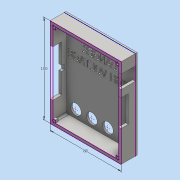
# Autodesk Inventor part: ATX Cover
Saved by Autodesk Inventor 2016 (Build 200138000, 138)
## iProperties
Created: 2016-08-04
Part Number: ATX Cover
Material: Generic
Document SubType Name: Modeling
Designer: Sam
Density: 1 g/cm^3
Appearance: Default
Author: Sam
Autodesk Inventor part; units mm, degrees
ref_plane "YZ Plane" through (0, 0, 0) normal (1, 0, 0) x (0, 1, 0)
ref_plane "XZ Plane" through (0, 0, 0) normal (0, 1, 0) x (-1, 0, 0)
ref_plane "XY Plane" through (0, 0, 0) normal (0, 0, 1) x (1, 0, 0)
sketch "Sketch1" plane through (0, 0, 0) normal (0, 1, 0) x (-1, 0, 0)
  line L0 (0, 0) -> (80, 0)
  line L1 (80, 0) -> (80, -100)
  line L2 (80, -100) -> (0, -100)
  line L3 (0, -100) -> (0, 0)
  line L4 (77, -97) -> (77, -3)
  line L5 (77, -3) -> (3, -3)
  line L6 (3, -3) -> (3, -97)
  line L7 (3, -97) -> (77, -97)
  line L8 (77, -3) -> (74, -3)
  line L9 (74, -3) -> (74, -6)
  line L10 (74, -6) -> (77, -6)
  line L11 (77, -6) -> (77, -3)
  line L12 (3, -3) -> (6, -3)
  line L13 (6, -3) -> (6, -6)
  line L14 (6, -6) -> (3, -6)
  line L15 (3, -6) -> (3, -3)
  line L16 (3, -97) -> (6, -97)
  line L17 (6, -97) -> (6, -94)
  line L18 (6, -94) -> (3, -94)
  line L19 (3, -94) -> (3, -97)
  line L20 (77, -97) -> (74, -97)
  line L21 (74, -97) -> (74, -94)
  line L22 (74, -94) -> (77, -94)
  line L23 (77, -94) -> (77, -97)
  point P0 (4, -4)
  point P1 (76, -4)
  point P2 (76, -96)
  point P3 (4, -96)
  dimension "d2" = 80
  dimension "d3" = 100
  constraints: 48 end point, 12 parallel, 6 perpendicular, 5 horizontal, 4 point on line, 3 other
  measures "d2" distance of L1.end L2.end
  measures "d3" distance of L0.end L1.end
extrude "Extrusion1" add sketch "Sketch1" along normal blind 16
extrude "Extrusion2" add sketch "Sketch1" along normal blind 3 contours L7 L21 L22 L4 | L10 L9 L5 L4 | L7 L6 L18 L17 | L13 L14 L6 L5
hole "Hole1" at (-4, 0, -4) at (-76, 0, -4) at (-76, 0, -96) at (-4, 0, -96) direction (0, 1, 0) diameter 3 end through all
sketch "Sketch2" plane through (0, 16, 0) normal (0, 1, 0) x (1, 0, 0)
  line L0 (-80, 0) -> (-80, 100) projected
  line L1 (-80, 0) -> (0, 0)
  line L2 (0, 0) -> (0, 100)
  line L3 (0, 100) -> (-80, 100)
  line L4 (-80, 100) -> (-80, 0)
  point P0 (-13, 89.5)
  point P1 (-31, 88)
  point P2 (-49, 88)
  point P3 (-67, 88)
  constraints: 8 end point, 2 parallel, 1 horizontal, 1 perpendicular
extrude "Extrusion3" add sketch "Sketch2" along normal blind 2
hole "Hole2" at (-67, 16, -88) at (-49, 16, -88) at (-31, 16, -88) at (-13, 16, -89.5) direction (0, 1, 0) diameter 12 end through all
sketch "Sketch3" plane through (0, 0, 0) normal (1, 0, 0) x (0, 0, -1)
  line L0 (94, 0) -> (6, 0) projected
  line L1 (5.118, 16) -> (94.882, 16) projected
  line L2 (12, 0) -> (27, 0)
  line L3 (27, 0) -> (27, 16)
  line L4 (27, 16) -> (12, 16)
  line L5 (12, 16) -> (12, 0)
  line L6 (35, 0) -> (65, 0)
  line L7 (65, 0) -> (65, 8)
  line L8 (65, 8) -> (35, 8)
  line L9 (35, 8) -> (35, 0)
  point P0 (0, 0)
  constraints: 16 end point, 4 parallel, 3 point on line, 2 horizontal, 2 perpendicular
extrude "Extrusion4" cut sketch "Sketch3" against normal blind 4
sketch "Sketch4" plane through (-80, 0, -100) normal (-1, 0, 0) x (0, 0, 1)
  line L0 (0, 0) -> (35, 0) projected
  line L1 (24, 0) -> (76, 0)
  line L2 (76, 0) -> (76, 10)
  line L3 (24, 10) -> (24, 0)
  line L4 (53, 10) -> (53, 13)
  line L5 (53, 13) -> (47, 13)
  line L6 (47, 13) -> (47, 10)
  line L7 (76, 10) -> (53, 10)
  line L8 (47, 10) -> (24, 10)
  point P0 (100, 0)
  constraints: 16 end point, 4 parallel, 1 horizontal, 1 perpendicular, 1 point on line
extrude "Extrusion5" cut sketch "Sketch4" against normal blind 4
sketch "Sketch5" plane through (0, 18, 0) normal (0, 1, 0) x (1, 0, 0)
  line L0 (0, 100) -> (-80, 100) projected
  line L1 (-80, 100) -> (-80, 0) projected
  line L2 (-80, 0) -> (0, 0) projected
  line L3 (0, 0) -> (0, 100) projected
  line L4 (-4, 20.3014) -> (-76, 20.3014) construction
  line L5 (-76, 20.3014) -> (-76, 40.6028) construction
  line L6 (-76, 40.6028) -> (-4, 40.6028) construction
  line L7 (-4, 40.6028) -> (-4, 20.3014) construction
  spline S0 degree 2 poles (-26.9997, 24.2223) (-26.9997, 25.2577) (-26.1604, 26.9241) (-25.4559, 27.3897) knots 0 0 0 1 2 2 2
  spline S1 degree 2 poles (-25.4559, 27.3897) (-24.88, 27.7511) (-23.6976, 27.9962) (-22.7786, 27.9962) knots 0 0 0 1 2 2 2
  line L8 (-22.7786, 27.9962) -> (-21.0387, 27.9962)
  line L9 (-21.0387, 27.9962) -> (-21.0387, 20.4362)
  line L10 (-21.0387, 20.4362) -> (-22.7603, 20.4362)
  spline S2 degree 2 poles (-22.7603, 20.4362) (-23.8263, 20.4362) (-25.0393, 20.7548) (-25.4681, 21.0366) knots 0 0 0 1 2 2 2
  spline S3 degree 2 poles (-25.4681, 21.0366) (-26.1972, 21.5206) (-26.9997, 23.1196) (-26.9997, 24.2223) knots 0 0 0 1 2 2 2
  spline S4 degree 2 poles (-25.9521, 24.2101) (-25.9521, 23.3401) (-25.3762, 22.1087) (-24.8065, 21.7595) knots 0 0 0 1 2 2 2
  spline S5 degree 2 poles (-24.8065, 21.7595) (-24.4021, 21.5206) (-23.4893, 21.3061) (-22.8093, 21.3061) knots 0 0 0 1 2 2 2
  line L11 (-22.8093, 21.3061) -> (-22.0435, 21.3061)
  line L12 (-22.0435, 21.3061) -> (-22.0435, 27.1262)
  line L13 (-22.0435, 27.1262) -> (-22.8093, 27.1262)
  spline S6 degree 2 poles (-22.8093, 27.1262) (-23.477, 27.1262) (-24.4879, 26.9118) (-24.8984, 26.6239) knots 0 0 0 1 2 2 2
  spline S7 degree 2 poles (-24.8984, 26.6239) (-25.4253, 26.2685) (-25.9521, 25.0923) (-25.9521, 24.2101) knots 0 0 0 1 2 2 2
  line L14 (-27.2754, 27.9962) -> (-29.824, 20.4362)
  line L15 (-29.824, 20.4362) -> (-31.0616, 20.4362)
  line L16 (-31.0616, 20.4362) -> (-33.6101, 27.9962)
  line L17 (-33.6101, 27.9962) -> (-32.5503, 27.9962)
  line L18 (-32.5503, 27.9962) -> (-31.8641, 25.8826)
  line L19 (-31.8641, 25.8826) -> (-28.9786, 25.8826)
  line L20 (-28.9786, 25.8826) -> (-28.2924, 27.9962)
  line L21 (-28.2924, 27.9962) -> (-27.2754, 27.9962)
  line L22 (-31.5884, 25.0249) -> (-30.4183, 21.4654)
  line L23 (-30.4183, 21.4654) -> (-29.2543, 25.0249)
  line L24 (-29.2543, 25.0249) -> (-31.5884, 25.0249)
  line L25 (-39.7366, 27.9962) -> (-38.6093, 27.9962)
  line L26 (-38.6093, 27.9962) -> (-35.2643, 21.4777)
  line L27 (-35.2643, 21.4777) -> (-35.2643, 27.9962)
  line L28 (-35.2643, 27.9962) -> (-34.3269, 27.9962)
  line L29 (-34.3269, 27.9962) -> (-34.3269, 20.4362)
  line L30 (-34.3269, 20.4362) -> (-35.7544, 20.4362)
  line L31 (-35.7544, 20.4362) -> (-38.7992, 26.4217)
  line L32 (-38.7992, 26.4217) -> (-38.7992, 20.4362)
  line L33 (-38.7992, 20.4362) -> (-39.7366, 20.4362)
  line L34 (-39.7366, 20.4362) -> (-39.7366, 27.9962)
  spline S8 degree 2 poles (-44.4355, 28.1432) (-43.633, 28.1432) (-42.3035, 27.6531) (-41.8257, 27.1569) knots 0 0 0 1 2 2 2
  spline S9 degree 2 poles (-41.8257, 27.1569) (-41.3478, 26.6545) (-40.8393, 25.1719) (-40.8393, 24.2101) knots 0 0 0 1 2 2 2
  spline S10 degree 2 poles (-40.8393, 24.2101) (-40.8393, 23.2972) (-41.3539, 21.8514) (-41.8318, 21.3368) knots 0 0 0 1 2 2 2
  spline S11 degree 2 poles (-41.8318, 21.3368) (-42.2913, 20.8405) (-43.6391, 20.3014) (-44.4417, 20.3014) knots 0 0 0 1 2 2 2
  spline S12 degree 2 poles (-44.4417, 20.3014) (-44.8276, 20.3014) (-45.526, 20.4117) (-45.8446, 20.5097) knots 0 0 0 1 2 2 2
  spline S13 degree 2 poles (-45.8446, 20.5097) (-46.1019, 20.5832) (-46.7268, 20.8528) (-46.9167, 20.9508) knots 0 0 0 1 2 2 2
  line L35 (-46.9167, 20.9508) -> (-46.9167, 22.1638)
  line L36 (-46.9167, 22.1638) -> (-46.831, 22.1638)
  spline S14 degree 2 poles (-46.831, 22.1638) (-46.641, 21.9984) (-46.2428, 21.6982) (-45.8752, 21.5267) knots 0 0 0 1 2 2 2
  spline S15 degree 2 poles (-45.8752, 21.5267) (-45.5689, 21.3735) (-44.7786, 21.1714) (-44.3253, 21.1714) knots 0 0 0 1 2 2 2
  spline S16 degree 2 poles (-44.3253, 21.1714) (-43.2347, 21.1714) (-41.8869, 22.8132) (-41.8869, 24.1794) knots 0 0 0 1 2 2 2
  spline S17 degree 2 poles (-41.8869, 24.1794) (-41.8869, 24.9391) (-42.2423, 26.0786) (-42.5792, 26.4707) knots 0 0 0 1 2 2 2
  spline S18 degree 2 poles (-42.5792, 26.4707) (-42.9039, 26.8628) (-43.8229, 27.2733) (-44.3988, 27.2733) knots 0 0 0 1 2 2 2
  spline S19 degree 2 poles (-44.3988, 27.2733) (-44.8215, 27.2733) (-45.6669, 27.1507) (-45.9549, 27.0282) knots 0 0 0 1 2 2 2
  line L37 (-45.9549, 27.0282) -> (-45.9549, 25.0739)
  line L38 (-45.9549, 25.0739) -> (-44.2027, 25.0739)
  line L39 (-44.2027, 25.0739) -> (-44.2027, 24.1917)
  line L40 (-44.2027, 24.1917) -> (-46.9474, 24.1917)
  line L41 (-46.9474, 24.1917) -> (-46.9474, 27.4938)
  spline S20 degree 2 poles (-46.9474, 27.4938) (-46.7574, 27.5796) (-46.108, 27.843) (-45.8324, 27.9227) knots 0 0 0 1 2 2 2
  spline S21 degree 2 poles (-45.8324, 27.9227) (-45.4586, 28.0329) (-44.8582, 28.1432) (-44.4355, 28.1432) knots 0 0 0 1 2 2 2
  line L42 (-48.2094, 27.9962) -> (-48.2094, 20.4362)
  line L43 (-48.2094, 20.4362) -> (-52.939, 20.4362)
  line L44 (-52.939, 20.4362) -> (-52.939, 21.3306)
  line L45 (-52.939, 21.3306) -> (-49.2141, 21.3306)
  line L46 (-49.2141, 21.3306) -> (-49.2141, 23.4014)
  line L47 (-49.2141, 23.4014) -> (-52.6878, 23.4014)
  line L48 (-52.6878, 23.4014) -> (-52.6878, 24.2958)
  line L49 (-52.6878, 24.2958) -> (-49.2141, 24.2958)
  line L50 (-49.2141, 24.2958) -> (-49.2141, 27.1017)
  line L51 (-49.2141, 27.1017) -> (-52.939, 27.1017)
  line L52 (-52.939, 27.1017) -> (-52.939, 27.9962)
  line L53 (-52.939, 27.9962) -> (-48.2094, 27.9962)
  line L54 (-59.8925, 27.9962) -> (-58.5876, 27.9962)
  line L55 (-58.5876, 27.9962) -> (-56.1983, 24.9881)
  line L56 (-56.1983, 24.9881) -> (-55.0465, 24.9881)
  line L57 (-55.0465, 24.9881) -> (-55.0465, 27.9962)
  line L58 (-55.0465, 27.9962) -> (-54.0418, 27.9962)
  line L59 (-54.0418, 27.9962) -> (-54.0418, 20.4362)
  line L60 (-54.0418, 20.4362) -> (-55.99, 20.4362)
  spline S22 degree 2 poles (-55.99, 20.4362) (-56.6394, 20.4362) (-57.5154, 20.5771) (-57.9136, 20.8344) knots 0 0 0 1 2 2 2
  spline S23 degree 2 poles (-57.9136, 20.8344) (-58.3119, 21.0917) (-58.7713, 21.8943) (-58.7713, 22.4885) knots 0 0 0 1 2 2 2
  spline S24 degree 2 poles (-58.7713, 22.4885) (-58.7713, 23.3156) (-57.9259, 24.4367) (-57.203, 24.7063) knots 0 0 0 1 2 2 2
  line L61 (-57.203, 24.7063) -> (-59.8925, 27.9962)
  spline S25 degree 2 poles (-57.7237, 22.5682) (-57.7237, 22.2374) (-57.4909, 21.7289) (-57.2459, 21.5635) knots 0 0 0 1 2 2 2
  spline S26 degree 2 poles (-57.2459, 21.5635) (-57.0314, 21.4225) (-56.4617, 21.3061) (-56.0451, 21.3061) knots 0 0 0 1 2 2 2
  line L62 (-56.0451, 21.3061) -> (-55.0465, 21.3061)
  line L63 (-55.0465, 21.3061) -> (-55.0465, 24.1488)
  line L64 (-55.0465, 24.1488) -> (-55.9287, 24.1488)
  spline S27 degree 2 poles (-55.9287, 24.1488) (-56.3637, 24.1488) (-57.0559, 23.9956) (-57.2949, 23.7567) knots 0 0 0 1 2 2 2
  spline S28 degree 2 poles (-57.2949, 23.7567) (-57.5154, 23.5484) (-57.7237, 22.9603) (-57.7237, 22.5682) knots 0 0 0 1 2 2 2
  line L65 (-10.293, 40.4435) -> (-9.2883, 40.4435)
  line L66 (-9.2883, 40.4435) -> (-9.2883, 36.7432)
  line L67 (-9.2883, 36.7432) -> (-5.8085, 36.7432)
  line L68 (-5.8085, 36.7432) -> (-5.8085, 40.4435)
  line L69 (-5.8085, 40.4435) -> (-4.8037, 40.4435)
  line L70 (-4.8037, 40.4435) -> (-4.8037, 32.8835)
  line L71 (-4.8037, 32.8835) -> (-5.8085, 32.8835)
  line L72 (-5.8085, 32.8835) -> (-5.8085, 35.8487)
  line L73 (-5.8085, 35.8487) -> (-9.2883, 35.8487)
  line L74 (-9.2883, 35.8487) -> (-9.2883, 32.8835)
  line L75 (-9.2883, 32.8835) -> (-10.293, 32.8835)
  line L76 (-10.293, 32.8835) -> (-10.293, 40.4435)
  line L77 (-14.459, 40.4435) -> (-11.5305, 40.4435)
  line L78 (-11.5305, 40.4435) -> (-11.5305, 39.6716)
  line L79 (-11.5305, 39.6716) -> (-12.4924, 39.6716)
  line L80 (-12.4924, 39.6716) -> (-12.4924, 33.6555)
  line L81 (-12.4924, 33.6555) -> (-11.5305, 33.6555)
  line L82 (-11.5305, 33.6555) -> (-11.5305, 32.8835)
  line L83 (-11.5305, 32.8835) -> (-14.459, 32.8835)
  line L84 (-14.459, 32.8835) -> (-14.459, 33.6555)
  line L85 (-14.459, 33.6555) -> (-13.4971, 33.6555)
  line L86 (-13.4971, 33.6555) -> (-13.4971, 39.6716)
  line L87 (-13.4971, 39.6716) -> (-14.459, 39.6716)
  line L88 (-14.459, 39.6716) -> (-14.459, 40.4435)
  spline S29 degree 2 poles (-18.87, 40.5906) (-18.0674, 40.5906) (-16.738, 40.1005) (-16.2601, 39.6042) knots 0 0 0 1 2 2 2
  spline S30 degree 2 poles (-16.2601, 39.6042) (-15.7823, 39.1018) (-15.2738, 37.6193) (-15.2738, 36.6574) knots 0 0 0 1 2 2 2
  spline S31 degree 2 poles (-15.2738, 36.6574) (-15.2738, 35.7446) (-15.7884, 34.2987) (-16.2663, 33.7841) knots 0 0 0 1 2 2 2
  spline S32 degree 2 poles (-16.2663, 33.7841) (-16.7257, 33.2879) (-18.0735, 32.7487) (-18.8761, 32.7487) knots 0 0 0 1 2 2 2
  spline S33 degree 2 poles (-18.8761, 32.7487) (-19.2621, 32.7487) (-19.9605, 32.859) (-20.2791, 32.957) knots 0 0 0 1 2 2 2
  spline S34 degree 2 poles (-20.2791, 32.957) (-20.5364, 33.0306) (-21.1613, 33.3001) (-21.3512, 33.3981) knots 0 0 0 1 2 2 2
  line L89 (-21.3512, 33.3981) -> (-21.3512, 34.6112)
  line L90 (-21.3512, 34.6112) -> (-21.2654, 34.6112)
  spline S35 degree 2 poles (-21.2654, 34.6112) (-21.0755, 34.4458) (-20.6773, 34.1456) (-20.3097, 33.974) knots 0 0 0 1 2 2 2
  spline S36 degree 2 poles (-20.3097, 33.974) (-20.0034, 33.8209) (-19.2131, 33.6187) (-18.7597, 33.6187) knots 0 0 0 1 2 2 2
  spline S37 degree 2 poles (-18.7597, 33.6187) (-17.6692, 33.6187) (-16.3214, 35.2606) (-16.3214, 36.6268) knots 0 0 0 1 2 2 2
  spline S38 degree 2 poles (-16.3214, 36.6268) (-16.3214, 37.3864) (-16.6767, 38.526) (-17.0137, 38.9181) knots 0 0 0 1 2 2 2
  spline S39 degree 2 poles (-17.0137, 38.9181) (-17.3384, 39.3101) (-18.2573, 39.7206) (-18.8332, 39.7206) knots 0 0 0 1 2 2 2
  spline S40 degree 2 poles (-18.8332, 39.7206) (-19.2559, 39.7206) (-20.1014, 39.5981) (-20.3893, 39.4756) knots 0 0 0 1 2 2 2
  line L91 (-20.3893, 39.4756) -> (-20.3893, 37.5212)
  line L92 (-20.3893, 37.5212) -> (-18.6372, 37.5212)
  line L93 (-18.6372, 37.5212) -> (-18.6372, 36.639)
  line L94 (-18.6372, 36.639) -> (-21.3818, 36.639)
  line L95 (-21.3818, 36.639) -> (-21.3818, 39.9412)
  spline S41 degree 2 poles (-21.3818, 39.9412) (-21.1919, 40.0269) (-20.5425, 40.2904) (-20.2668, 40.37) knots 0 0 0 1 2 2 2
  spline S42 degree 2 poles (-20.2668, 40.37) (-19.8931, 40.4803) (-19.2927, 40.5906) (-18.87, 40.5906) knots 0 0 0 1 2 2 2
  line L96 (-28.1331, 40.4435) -> (-27.1284, 40.4435)
  line L97 (-27.1284, 40.4435) -> (-27.1284, 36.7432)
  line L98 (-27.1284, 36.7432) -> (-23.6486, 36.7432)
  line L99 (-23.6486, 36.7432) -> (-23.6486, 40.4435)
  line L100 (-23.6486, 40.4435) -> (-22.6439, 40.4435)
  line L101 (-22.6439, 40.4435) -> (-22.6439, 32.8835)
  line L102 (-22.6439, 32.8835) -> (-23.6486, 32.8835)
  line L103 (-23.6486, 32.8835) -> (-23.6486, 35.8487)
  line L104 (-23.6486, 35.8487) -> (-27.1284, 35.8487)
  line L105 (-27.1284, 35.8487) -> (-27.1284, 32.8835)
  line L106 (-27.1284, 32.8835) -> (-28.1331, 32.8835)
  line L107 (-28.1331, 32.8835) -> (-28.1331, 40.4435)
  line L108 (-38.3949, 32.8835) -> (-35.7912, 40.4435)
  line L109 (-35.7912, 40.4435) -> (-34.7068, 40.4435)
  line L110 (-34.7068, 40.4435) -> (-32.103, 32.8835)
  line L111 (-32.103, 32.8835) -> (-33.1813, 32.8835)
  line L112 (-33.1813, 32.8835) -> (-35.2765, 39.1631)
  line L113 (-35.2765, 39.1631) -> (-37.3718, 32.8835)
  line L114 (-37.3718, 32.8835) -> (-38.3949, 32.8835)
  spline S43 degree 2 poles (-44.4662, 33.7474) (-44.895, 34.2497) (-45.3729, 35.7201) (-45.3729, 36.6635) knots 0 0 0 1 2 2 2
  spline S44 degree 2 poles (-45.3729, 36.6635) (-45.3729, 37.5825) (-44.9073, 39.0712) (-44.4662, 39.5736) knots 0 0 0 1 2 2 2
  spline S45 degree 2 poles (-44.4662, 39.5736) (-44.0006, 40.1005) (-42.7691, 40.6028) (-42.0278, 40.6028) knots 0 0 0 1 2 2 2
  spline S46 degree 2 poles (-42.0278, 40.6028) (-41.262, 40.6028) (-40.0368, 40.0821) (-39.5895, 39.5736) knots 0 0 0 1 2 2 2
  spline S47 degree 2 poles (-39.5895, 39.5736) (-39.1546, 39.0712) (-38.6889, 37.5947) (-38.6889, 36.6635) knots 0 0 0 1 2 2 2
  spline S48 degree 2 poles (-38.6889, 36.6635) (-38.6889, 35.7139) (-39.1607, 34.2681) (-39.5957, 33.7474) knots 0 0 0 1 2 2 2
  spline S49 degree 2 poles (-39.5957, 33.7474) (-40.0368, 33.245) (-41.2682, 32.7242) (-42.0278, 32.7242) knots 0 0 0 1 2 2 2
  spline S50 degree 2 poles (-42.0278, 32.7242) (-42.7998, 32.7242) (-44.0373, 33.2634) (-44.4662, 33.7474) knots 0 0 0 1 2 2 2
  spline S51 degree 2 poles (-44.3253, 36.6635) (-44.3253, 35.9161) (-44.0006, 34.7582) (-43.7065, 34.3784) knots 0 0 0 1 2 2 2
  spline S52 degree 2 poles (-43.7065, 34.3784) (-43.4063, 33.9863) (-42.5608, 33.5942) (-42.034, 33.5942) knots 0 0 0 1 2 2 2
  spline S53 degree 2 poles (-42.034, 33.5942) (-41.4887, 33.5942) (-40.6678, 33.974) (-40.3553, 34.3784) knots 0 0 0 1 2 2 2
  spline S54 degree 2 poles (-40.3553, 34.3784) (-40.0551, 34.7643) (-39.7366, 35.9284) (-39.7366, 36.6635) knots 0 0 0 1 2 2 2
  spline S55 degree 2 poles (-39.7366, 36.6635) (-39.7366, 38.1523) (-40.9864, 39.7329) (-42.034, 39.7329) knots 0 0 0 1 2 2 2
  spline S56 degree 2 poles (-42.034, 39.7329) (-43.0816, 39.7329) (-44.3253, 38.1523) (-44.3253, 36.6635) knots 0 0 0 1 2 2 2
  line L115 (-50.856, 40.4435) -> (-46.4756, 40.4435)
  line L116 (-46.4756, 40.4435) -> (-46.4756, 32.8835)
  line L117 (-46.4756, 32.8835) -> (-47.4804, 32.8835)
  line L118 (-47.4804, 32.8835) -> (-47.4804, 39.5491)
  line L119 (-47.4804, 39.5491) -> (-50.856, 39.5491)
  line L120 (-50.856, 39.5491) -> (-50.856, 40.4435)
  line L121 (-53.4107, 40.4435) -> (-53.4107, 33.778)
  line L122 (-53.4107, 33.778) -> (-50.8744, 33.778)
  line L123 (-50.8744, 33.778) -> (-50.8744, 32.8835)
  line L124 (-50.8744, 32.8835) -> (-56.9518, 32.8835)
  line L125 (-56.9518, 32.8835) -> (-56.9518, 33.778)
  line L126 (-56.9518, 33.778) -> (-54.4155, 33.778)
  line L127 (-54.4155, 33.778) -> (-54.4155, 40.4435)
  line L128 (-54.4155, 40.4435) -> (-53.4107, 40.4435)
  line L129 (-56.9028, 40.4435) -> (-59.4514, 32.8835)
  line L130 (-59.4514, 32.8835) -> (-60.6889, 32.8835)
  line L131 (-60.6889, 32.8835) -> (-63.2375, 40.4435)
  line L132 (-63.2375, 40.4435) -> (-62.1776, 40.4435)
  line L133 (-62.1776, 40.4435) -> (-61.4915, 38.3299)
  line L134 (-61.4915, 38.3299) -> (-58.6059, 38.3299)
  line L135 (-58.6059, 38.3299) -> (-57.9198, 40.4435)
  line L136 (-57.9198, 40.4435) -> (-56.9028, 40.4435)
  line L137 (-61.2158, 37.4722) -> (-60.0456, 33.9128)
  line L138 (-60.0456, 33.9128) -> (-58.8816, 37.4722)
  line L139 (-58.8816, 37.4722) -> (-61.2158, 37.4722)
  spline S57 degree 2 poles (-67.1217, 40.5906) (-66.3191, 40.5906) (-64.9897, 40.1005) (-64.5118, 39.6042) knots 0 0 0 1 2 2 2
  spline S58 degree 2 poles (-64.5118, 39.6042) (-64.0339, 39.1018) (-63.5254, 37.6193) (-63.5254, 36.6574) knots 0 0 0 1 2 2 2
  spline S59 degree 2 poles (-63.5254, 36.6574) (-63.5254, 35.7446) (-64.0401, 34.2987) (-64.5179, 33.7841) knots 0 0 0 1 2 2 2
  spline S60 degree 2 poles (-64.5179, 33.7841) (-64.9774, 33.2879) (-66.3252, 32.7487) (-67.1278, 32.7487) knots 0 0 0 1 2 2 2
  spline S61 degree 2 poles (-67.1278, 32.7487) (-67.5137, 32.7487) (-68.2122, 32.859) (-68.5307, 32.957) knots 0 0 0 1 2 2 2
  spline S62 degree 2 poles (-68.5307, 32.957) (-68.788, 33.0306) (-69.4129, 33.3001) (-69.6029, 33.3981) knots 0 0 0 1 2 2 2
  line L140 (-69.6029, 33.3981) -> (-69.6029, 34.6112)
  line L141 (-69.6029, 34.6112) -> (-69.5171, 34.6112)
  spline S63 degree 2 poles (-69.5171, 34.6112) (-69.3272, 34.4458) (-68.9289, 34.1456) (-68.5614, 33.974) knots 0 0 0 1 2 2 2
  spline S64 degree 2 poles (-68.5614, 33.974) (-68.255, 33.8209) (-67.4647, 33.6187) (-67.0114, 33.6187) knots 0 0 0 1 2 2 2
  spline S65 degree 2 poles (-67.0114, 33.6187) (-65.9209, 33.6187) (-64.5731, 35.2606) (-64.5731, 36.6268) knots 0 0 0 1 2 2 2
  spline S66 degree 2 poles (-64.5731, 36.6268) (-64.5731, 37.3864) (-64.9284, 38.526) (-65.2654, 38.9181) knots 0 0 0 1 2 2 2
  spline S67 degree 2 poles (-65.2654, 38.9181) (-65.5901, 39.3101) (-66.509, 39.7206) (-67.0849, 39.7206) knots 0 0 0 1 2 2 2
  spline S68 degree 2 poles (-67.0849, 39.7206) (-67.5076, 39.7206) (-68.3531, 39.5981) (-68.641, 39.4756) knots 0 0 0 1 2 2 2
  line L142 (-68.641, 39.4756) -> (-68.641, 37.5212)
  line L143 (-68.641, 37.5212) -> (-66.8889, 37.5212)
  line L144 (-66.8889, 37.5212) -> (-66.8889, 36.639)
  line L145 (-66.8889, 36.639) -> (-69.6335, 36.639)
  line L146 (-69.6335, 36.639) -> (-69.6335, 39.9412)
  spline S69 degree 2 poles (-69.6335, 39.9412) (-69.4436, 40.0269) (-68.7942, 40.2904) (-68.5185, 40.37) knots 0 0 0 1 2 2 2
  spline S70 degree 2 poles (-68.5185, 40.37) (-68.1448, 40.4803) (-67.5444, 40.5906) (-67.1217, 40.5906) knots 0 0 0 1 2 2 2
  line L147 (-70.8955, 40.4435) -> (-70.8955, 32.8835)
  line L148 (-70.8955, 32.8835) -> (-75.6251, 32.8835)
  line L149 (-75.6251, 32.8835) -> (-75.6251, 33.778)
  line L150 (-75.6251, 33.778) -> (-71.9003, 33.778)
  line L151 (-71.9003, 33.778) -> (-71.9003, 35.8487)
  line L152 (-71.9003, 35.8487) -> (-75.3739, 35.8487)
  line L153 (-75.3739, 35.8487) -> (-75.3739, 36.7432)
  line L154 (-75.3739, 36.7432) -> (-71.9003, 36.7432)
  line L155 (-71.9003, 36.7432) -> (-71.9003, 39.5491)
  line L156 (-71.9003, 39.5491) -> (-75.6251, 39.5491)
  line L157 (-75.6251, 39.5491) -> (-75.6251, 40.4435)
  line L158 (-75.6251, 40.4435) -> (-70.8955, 40.4435)
  dimension "d39" = 4
  dimension "d40" = 4
  constraints: 2 other
  measures "d39" distance between parallel lines of L1 L5
  measures "d40" distance between parallel lines of L3 L7
extrude "Extrusion6" cut sketch "Sketch5" against normal blind 4 contours S0 S1 L8 L9 L10 S2 S3 | L14 L15 L16 L17 L18 L19 L20 L21 | L25 L26 L27 L28 L29 L30 L31 L32 L33 L34 | S8 S9 S10 S11 S12 S13 L35 L36 S14 S15 S16 S17 S18 S19 L37 L38 L39 L40 L41 S20 S21 | L42 L43 L44 L45 L46 L47 L48 L49 L50 L51 L52 L53 | L54 L55 L56 L57 L58 L59 L60 S22 S23 S24 L61 | L65 L66 L67 L68 L69 L70 L71 L72 L73 L74 L75 L76 | L77 L78 L79 L80 L81 L82 L83 L84 L85 L86 L87 L88 | S29 S30 S31 S32 S33 S34 L89 L90 S35 S36 S37 S38 S39 S40 L91 L92 L93 L94 L95 S41 S42 | L96 L97 L98 L99 L100 L101 L102 L103 L104 L105 L106 L107 | L108 L109 L110 L111 L112 L113 L114 | S43 S44 S45 S46 S47 S48 S49 S50 | L115 L116 L117 L118 L119 L120 | L121 L122 L123 L124 L125 L126 L127 L128 | L129 L130 L131 L132 L133 L134 L135 L136 | S57 S58 S59 S60 S61 S62 L140 L141 S63 S64 S65 S66 S67 S68 L142 L143 L144 L145 L146 S69 S70 | L147 L148 L149 L150 L151 L152 L153 L154 L155 L156 L157 L158
body "Solid1"
